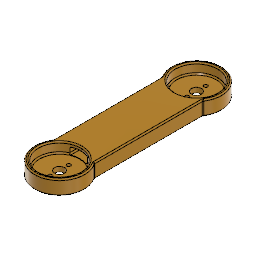
Braco_1_v4 (Autodesk Fusion 360 design; units mm, degrees)
Autodesk Fusion 360 part; units mm, degrees
sketch "Sketch1" plane through (0, 0, 0) normal (0, 0, 1) x (1, 0, 0)
  line L0 (33, 11.3027) -> (33, 98.6973)
  line L1 (0, 98.6973) -> (0, 11.3027)
  line L2 (16.5, 121.9181) -> (16.5, -40) construction
  arc A0 (0, 11.3027) -> (33, 11.3027) centre (16.5, 0) ccw
  arc A1 (33, 98.6973) -> (0, 98.6973) centre (16.5, 110) ccw
  circle A2 centre (16.5, 110) radius 17
  circle A3 centre (16.5, 0) radius 17
  circle A4 centre (16.5, 0) radius 4
  circle A5 centre (16.5, 110) radius 4
  circle A6 centre (16.5, 117.5) radius 1.5
  line L3 (28, 110) -> (2, 110) construction
  circle A7 centre (16.5, 102.5) radius 1.5
  circle A8 centre (16.5, 7.5) radius 1.5
  line L4 (6, 0) -> (29, 0) construction
  circle A9 centre (16.5, -7.5) radius 1.5
  dimension "d3" = 16.5
  dimension "d4" = 40
  dimension "d5" = 40
  dimension "d6" = 34
  dimension "d7" = 34
  dimension "d13" = 87.3947
  dimension "d14" = 33
  dimension "d15" = 8
  dimension "d16" = 8
  dimension "d17" = 3
  dimension "d18" = 7.5
  dimension "d19" = 3
  dimension "d20" = 7.5
  constraint vertical L0
  constraint vertical L1
  constraint concentric A1 A2
  constraint concentric A0 A3
  constraint concentric A3 A4
  constraint concentric A2 A5
  constraint coincident L2 A6.centre
  constraint horizontal L3
  constraint symmetric A6 L3 A7
  constraint coincident L2 A8.centre
  constraint perpendicular L2 L4
  constraint symmetric A8 L4 A9
  measures "d3" distance of L0 L2
  measures "d4" diameter of A1
  measures "d5" diameter of A0
  measures "d6" diameter of A2
  measures "d7" diameter of A3
  measures "d13" distance of L1.start L1.end
  measures "d14" distance of L0 L1
  measures "d15" diameter of A4
  measures "d16" diameter of A5
  measures "d17" diameter of A6
  measures "d18" distance of A1.centre A6.centre
  measures "d19" diameter of A8
  measures "d20" distance of A0.centre A8.centre
extrude "Extrude1" add sketch "Sketch1" along normal blind 12 contours L0 L1 A0 A1 | A2 | A3 | A4 | A5 | A6 | A7 | A8 | A9
extrude "Extrude2" cut sketch "Sketch1" against normal blind 8 from surface at 12 contours A2 | A3 | A4 | A5 | A6 | A7 | A8 | A9
extrude "Extrude3" cut sketch "Sketch1" along normal blind 20 contours A4 | A5 | A6 | A7 | A8 | A9
sketch "Sketch2" plane through (0, 0, 0) normal (0, 1, 0) x (1, 0, 0)
  line L0 (22.4729, -9.1691) -> (10.4729, -9.1691)
  line L1 (9.4729, -8.1691) -> (9.4729, -5.1691)
  line L2 (10.4729, -4.1691) -> (22.4729, -4.1691)
  line L3 (23.4729, -5.1691) -> (23.4729, -8.1691)
  line L4 (36.4729, -0.026) -> (36.4729, -8.5)
  line L5 (-3.434, -0.0044) -> (-3.434, -9.697)
  arc A0 (9.4729, -8.1691) -> (10.4729, -9.1691) centre (10.4729, -8.1691) ccw
  arc A1 (10.4729, -4.1691) -> (9.4729, -5.1691) centre (10.4729, -5.1691) ccw
  arc A2 (22.4729, -9.1691) -> (23.4729, -8.1691) centre (22.4729, -8.1691) ccw
  arc A3 (23.4729, -5.1691) -> (22.4729, -4.1691) centre (22.4729, -5.1691) ccw
  point P0 (9.4729, -9.1691)
  point P1 (9.4729, -4.1691)
  dimension "d25" = 5
  dimension "d26" = 1
  dimension "d27" = 1
  constraint horizontal L0
  constraint vertical L1
  constraint horizontal L2
  constraint vertical L3
  constraint vertical L4
  constraint vertical L5
  constraint coincident P0 L0
  constraint coincident P0 L1
  constraint tangent L0 A0
  constraint tangent L1 A0
  constraint coincident P1 L1
  constraint coincident P1 L2
  constraint tangent L1 A1
  constraint tangent L2 A1
  constraint tangent L0 A2
  constraint tangent L3 A2
  constraint equal A1 A2
  constraint tangent L2 A3
  constraint tangent L3 A3
  constraint equal A1 A3
  measures "d25" distance of P0 P1
  measures "d26" radius of A0
  measures "d27" radius of A1
extrude "Extrude4" cut sketch "Sketch2" along normal blind 110
fillet "Fillet1" radius 1 6 edges at (33, 55, 12) (16.5, -20, 12) (0, 55, 12) (16.5, 130, 12) (0.6504, 6.1475, 12) (0.6504, 116.1475, 12)
fillet "Fillet2" radius 1 4 edges at (33, 55, 0) (0, 55, 0) (16.5, 130, 0) (16.5, -20, 0)
chamfer "Chamfer1" distance 1 angle 45 1 edges at (0.6504, 6.1475, 4)
chamfer "Chamfer2" distance 1 angle 45 1 edges at (0.6504, 116.1475, 4)
chamfer "Chamfer3" distance 0.5 angle 45 3 edges at (33, 11.3027, 6) (32.6994, 11.2092, 11.7147) (32.6994, 11.2092, 0.2853)
chamfer "Chamfer4" distance 0.5 angle 45 3 edges at (0, 11.3027, 6) (0.3006, 11.2092, 11.7147) (0.3006, 11.2092, 0.2853)
chamfer "Chamfer5" distance 0.5 angle 45 3 edges at (0, 98.6973, 6) (0.3006, 98.7908, 11.7147) (0.3006, 98.7908, 0.2853)
chamfer "Chamfer6" distance 0.5 angle 45 3 edges at (33, 98.6973, 6) (32.6994, 98.7908, 11.7147) (32.6994, 98.7908, 0.2853)
component "haste 1" placed x (1, 0, 0) y (0, 1, 0) z (0, 0, 1) at (0, 0, 0)
